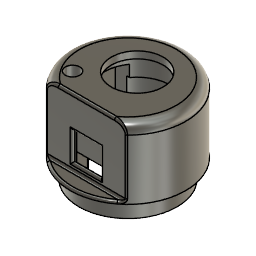
OpenTholoMetriV1 (Autodesk Fusion 360 design; units mm, degrees)
Autodesk Fusion 360 part; units mm, degrees
note: some values were not read from the file. Chosen so that the rebuilt part matches the saved one: which face or edge a step refers to; which sketch regions a step uses.
sketch "Sketch1" plane through (0, 0, 0) normal (0, 0, 1) x (1, 0, 0)
  circle A0 centre (0, 0) radius 21.25
  circle A1 centre (0, 0) radius 25
  dimension "d1" = 42.5
  dimension "d2" = 50
  constraint coincident A0.centre A1.centre
  constraint concentric A0 A1
  measures "d1" diameter of A0
  measures "d2" diameter of A1
sketch "Sketch2" plane through (0, 0, 0) normal (0, 0, 1) x (1, 0, 0)
  line L0 (-8.25, -14) -> (8.25, -14)
  line L1 (8.25, -14) -> (8.25, -17)
  line L2 (8.25, -17) -> (-8.25, -17)
  line L3 (-8.25, -17) -> (-8.25, -14)
  line L4 (-7, -17) -> (7, -17)
  line L5 (-10, -14) -> (10, -14)
  line L6 (10, -14) -> (10, 14)
  line L7 (10, 14) -> (-10, 14)
  line L8 (-10, 14) -> (-10, -14)
  dimension "d7" = 16.5
  dimension "d8" = 3
  dimension "d9" = 14
  dimension "d11" = 20
  dimension "d12" = 28
  constraint horizontal L0
  constraint vertical L1
  constraint horizontal L2
  constraint vertical L3
  constraint horizontal L4
  constraint coincident L2 L4.start
  constraint horizontal L5
  constraint vertical L6
  constraint horizontal L7
  constraint vertical L8
  constraint coincident L0 L5.start
  measures "d7" distance of L0.start L0.end
  measures "d8" distance of L0.start L2.end
  measures "d9" distance of L4.start L4.end
  measures "d11" distance of L5.start L5.end
  measures "d12" distance of L5.start L7.end
extrude "Extrude1" add sketch "Sketch1" along normal blind 38 contours A0 | A1
extrude "Extrude2" cut sketch "Sketch1" along normal blind 8
extrude "Extrude3" cut sketch "Sketch2" along normal blind 15
extrude "Extrude4" cut sketch "Sketch2" along normal blind 33 contours L0 L1 L2 L3 L4 L5
sketch "Sketch3" plane through (0, -18, 0) normal (0, 1, 0) x (-1, 0, 0)
  line L0 (-7, 0) -> (7, 0)
  line L1 (7, 0) -> (7, 33)
  line L2 (7, 33) -> (-7, 33)
  line L3 (-7, 33) -> (-7, 0)
  line L4 (-6, 12) -> (6, 12)
  line L5 (6, 12) -> (6, 24)
  line L6 (6, 24) -> (-6, 24)
  line L7 (-6, 24) -> (-6, 12)
  dimension "d17" = 12
  dimension "d18" = 12
  constraint horizontal L4
  constraint vertical L5
  constraint horizontal L6
  constraint vertical L7
  measures "d17" distance of L4.start L4.end
  measures "d18" distance of L4.start L6.end
extrude "Extrude5" cut sketch "Sketch3" against normal blind 7 contours L4 L5 L6 L7
extrude "Extrude6" cut sketch "Sketch2" along normal blind 20 contours L0 L5 L6 L7 L8
extrude "Extrude7" cut sketch "Sketch2" along normal blind 25 contours L0 L5 L6 L7 L8
fillet "Fillet1" radius 4 1 edges at (-23.3082, -9.0404, 38)
sketch "Sketch6" plane through (-6, 0, 0) normal (1, 0, 0) x (0, 1, 0)
  line L0 (-24.2693, 24) -> (-24.2693, 12)
  line L1 (-24.2693, 12) -> (-18, 12)
  line L2 (-18, 24) -> (-24.2693, 24)
  line L3 (-25, 25, -3) -> (-18.0683, 25, -3)
  line L4 (-18.0683, 25, -3) -> (-18.0683, 11, -3)
  line L5 (-18.0683, 11, -3) -> (-25, 11, -3)
  line L6 (-25, 11, -3) -> (-25, 25, -3)
  line L7 (-18, 12) -> (-18, 24)
sketch "Sketch6 (curves -3 mm off its plane)" plane through (-9, 0, 0) normal (1, 0, 0) x (0, 1, 0)
  line L0 (-25, 25) -> (-18.0683, 25)
  line L1 (-18.0683, 25) -> (-18.0683, 11)
  line L2 (-18.0683, 11) -> (-25, 11)
  line L3 (-25, 11) -> (-25, 25)
extrude "Extrude8" cut sketch "Sketch6 (curves -3 mm off its plane)" along normal blind 20
sketch "Sketch8" plane through (0, 0, 0) normal (0, 0, 1) x (1, 0, 0)
  circle A0 centre (0, 4) radius 11.25
  circle A1 centre (0, 4) radius 14.25
  line L0 (-17.75, 4) -> (-17.75, 12.25)
  line L1 (-17.7496, 4) -> (-17.7496, -4.25)
  line L2 (-17.7496, -4.25) -> (0, -4.25)
  line L3 (-17.75, 12.25) -> (0, 12.25)
  circle A2 centre (-14.3795, -9.638) radius 3.15
  line L4 (17.75, 12.25) -> (0, 12.25)
  line L5 (17.75, 3) -> (17.75, 12.25)
  line L6 (17.7496, 4) -> (17.7496, -4.25)
  line L7 (17.7496, -4.25) -> (0, -4.25)
  line L8 (-17.7496, -4.25) -> (17.75, -4.25)
  line L9 (17.75, -4.25) -> (17.75, 12.25)
  line L10 (17.75, 12.25) -> (-17.7496, 12.25)
  line L11 (-17.7496, 12.25) -> (-17.7496, -4.25)
  circle A3 centre (0, 4) radius 15.25
  dimension "d33" = 22.5
  dimension "d37" = 28.5
  dimension "d40" = 6.3
  dimension "d47" = 35.4992
  dimension "d50" = 30.5
  constraint concentric A0 A1
  constraint horizontal L8
  constraint vertical L9
  constraint horizontal L10
  constraint vertical L11
  constraint concentric A0 A3
  measures "d33" diameter of A0
  measures "d37" diameter of A1
  measures "d40" diameter of A2
  measures "d47" distance of L1 L6
  measures "d50" diameter of A3
extrude "Extrude11" cut sketch "Sketch8" along normal blind 76 contours A2
extrude "Extrude12" cut sketch "Sketch8" along normal blind 121 contours A0 L2 L3 L4 L7 L8 L10 | A0 L3 L4 L10 | A0 L2 L7 L8
extrude "Extrude13" cut sketch "Sketch8" along normal blind 35 contours A0 A1 L4 L7 L8 L10 | A0 L3 L4 L10 | A0 A1 L3 L4 L10 | A0 A1 L2 L7 L8 | A0 A1 L2 L3 L8 L10
extrude "Extrude15" cut sketch "Sketch8" along normal blind 26 contours A1 L4 L7 L8 L10 A3 | A1 L3 L4 L10 A3 | A1 L2 L7 L8 A3 | A1 L2 L3 L8 L10 A3
extrude "Extrude14" cut sketch "Sketch8" along normal blind 31 contours A0 A1 L4 L7 L8 L10 | A0 A1 L2 L3 L8 L10 | A1 L4 L7 L8 L10 A3 | A1 L2 L3 L8 L10 A3 | L4 L5 L6 L7 L8 L9 L10 A3 | L0 L1 L2 L3 L8 L10 L11 A3
extrude "Extrude18" cut 1 faces at (-9, -19.8201, 15.6667) along direction (1, 0, 0) blind 36
extrude "Extrude19" cut 1 faces at (-9, -19.8201, 15.6667) along direction (-1, 0, 0) blind 17
extrude "Extrude20" add 1 faces at (0, -13.0833, 25) along direction (0, 0, -1) blind 10
extrude "Extrude21" cut 1 faces at (2, -18, 20) along direction (0, 1, 0) blind 3
extrude "Extrude22" cut 1 faces at (1.5595, -22.4447, 25) along direction (0, 0, 1) blind 14
extrude "Extrude23" cut 1 faces at (-2.61, -20.9377, 11) along direction (0, 0, -1) blind 2
fillet "Fillet2" radius 1 2 faces at (-2, -18.0683, 33.3333) (-2.61, -20.9377, 9)
extrude "Extrude24" add 1 faces at (0, -13.0833, 15) along direction (0, 0, -1) blind 2
extrude "Extrude25" add 1 faces at (2.3333, -15, 33) along direction (0, 0, -1) blind 4
